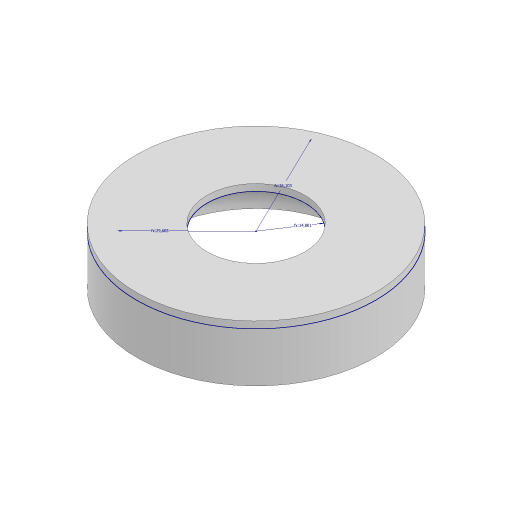
# Autodesk Inventor part: Korpus 2
Saved by Autodesk Inventor 2024 (Build 280153000, 153)
## iProperties
Created: 2024-12-22
Part Number: Korpus 2
Material: Ogólny
Document SubType Name: Modeling
Designer: Wicek
Density: 1 g/cm^3
Appearance: Domyślna
Author: Wicek
Autodesk Inventor part; units mm, degrees
ref_plane "YZ Plane" through (0, 0, 0) normal (1, 0, 0) x (0, 1, 0)
ref_plane "XZ Plane" through (0, 0, 0) normal (0, 1, 0) x (-1, 0, 0)
ref_plane "XY Plane" through (0, 0, 0) normal (0, 0, 1) x (1, 0, 0)
sketch "Szkic1" plane through (0, 0, 0) normal (0, 1, 0) x (-1, 0, 0)
  circle A0 centre (0, 0) radius 36.1028
  circle A1 centre (0, 0) radius 29.6028
  circle A2 centre (0, 0) radius 14.8014
  dimension "d16" = 36.1028
  dimension "d23" = 29.6028
  dimension "d28" = 14.8014
  constraints: 3 centre point, 3 coincident
  measures "d16" radius of A0
  measures "d23" radius of A1
  measures "d28" radius of A2
extrude "Wyciągnięcie proste1" add sketch "Szkic1" along normal blind 2 contours A0 | A1
extrude "Wyciągnięcie proste2" add sketch "Szkic1" against normal blind 15 contours A0
equation "\"d16\" = Rr + R + h2"
equation "\"d23\" = R"
equation "\"d28\" = 0.5 * R"
equation "\"d29\" = h1"
equation "\"Lrz\" = 11"
equation "\"Lrw\" = 4"
equation "\"Lh\" = 7"
equation "\"Rr\" = 1.5"
equation "\"R1\" = 5"
equation "\"h1\" = 2"
equation "\"h2\" = 5"
equation "\"E1\" = 0.5 * Rr"
equation "\"silnik_rw\" = 2.5"
equation "\"silnik_r_wypust\" = Lrz"
equation "\"silnik_d_srub\" = 31"
equation "\"dwr1\" = -0.25 * Rr + 0.25 * R - 0.25 * Lrz"
equation "\"dwr2\" = 0.5 * Lrz + 0.5 * R"
equation "\"dwr\" = R"
equation "\"R\" = 29.602819"
